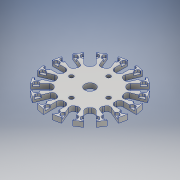
# Autodesk Inventor part: plate1_3mm_m6collet
Saved by Autodesk Inventor 2018 (Build 220112000, 112)
## iProperties
Created: 2017-08-17
Part Number: plate1_3mm_m6collet
Material: Aluminum 6061
Document SubType Name: Modeling
Designer: steve
Density: 2.7 g/cm^3
Appearance: Aluminum - Flat
Mass: 8.83202 g
Surface Area: 37.957 cm^2
Volume: 3.27112 cm^3
Author: steve
Autodesk Inventor part; units mm, degrees
note: some values were not read from the file. Chosen so that the rebuilt part matches the saved one: direction of "Hole3".
ref_plane "YZ Plane" through (0, 0, 0) normal (1, 0, 0) x (0, 1, 0)
ref_plane "XZ Plane" through (0, 0, 0) normal (0, 1, 0) x (-1, 0, 0)
ref_plane "XY Plane" through (0, 0, 0) normal (0, 0, 1) x (1, 0, 0)
sketch "Sketch1" plane through (0, 0, 0) normal (0, 0, 1) x (1, 0, 0)
  circle A0 centre (0, 0) radius 25
  dimension "wheel_border" = 50
  constraints: 1 centre point, 1 coincident
  measures "wheel_border" diameter of A0
extrude "Extrusion1" add sketch "Sketch1" along normal blind 3
sketch "Sketch4" plane through (0, 0, 3) normal (0, 0, 1) x (1, 0, 0)
  line L0 (-35, 0) -> (35, 0) construction
  line L1 (0, -35) -> (0, 35) construction
  line L2 (-11.282, 25) -> (10.768, 25) construction
  line L3 (-11.9075, 22.5) -> (11.2763, 22.5) construction
  circle A0 centre (0, 0) radius 25 construction
  line L4 (4.075, 20.9625) -> (-4.075, 20.9625) construction
  line L5 (-4.075, 20.9625) -> (-4.075, 24.0375) construction
  line L6 (-4.075, 24.0375) -> (4.075, 24.0375) construction
  line L7 (4.075, 24.0375) -> (4.075, 20.9625) construction
  line L8 (4.075, 20.9625) -> (-4.075, 24.0375) construction
  line L9 (-4.075, 20.9625) -> (4.075, 24.0375) construction
  line L10 (4.075, 20.9625) -> (-4.075, 20.9625)
  line L11 (-4.075, 20.9625) -> (-4.075, 24.0375)
  line L12 (-4.075, 24.0375) -> (4.075, 24.0375)
  line L13 (4.075, 24.0375) -> (4.075, 20.9625)
  line L14 (4.075, 20.9625) -> (-4.075, 24.0375) construction
  line L15 (-4.075, 20.9625) -> (4.075, 24.0375) construction
  point P0 (0, 22.5)
  dimension "d23" = 2.5
  dimension "d24" = 3.075
  dimension "d25" = 8.15
  constraints: 28 end point, 4 horizontal, 4 midpoint, 4 parallel, 2 perpendicular, 2 point on line, 1 tangent
  measures "d23" distance between parallel lines of L3 L2
  measures "d24" distance of L6.end L4.start
  measures "d25" distance of L4.start L4.end
extrude "Extrusion4" cut sketch "Sketch4" against normal blind 1.5
sketch "Sketch5" plane through (0, 0, 3) normal (0, 0, 1) x (1, 0, 0)
  line L0 (-4.075, 20.9625) -> (-4.075, 24.0375) construction
  line L1 (4.075, 20.9625) -> (-4.075, 20.9625) construction
  line L2 (4.075, 24.0375) -> (4.075, 20.9625) construction
  line L3 (-4.075, 24.0375) -> (4.075, 24.0375) construction
  line L4 (-35, 0) -> (35, 0) construction
  line L5 (0, -36.2) -> (0, 42.2) construction
  line L6 (-4.075, 22.5) -> (4.075, 22.5) construction
  line L7 (4.075, 24.0375) -> (4.075, 20.9625) construction
  line L8 (2.575, 15) -> (-2.575, 15)
  line L9 (-2.575, 15) -> (-2.575, 30)
  line L10 (-2.575, 30) -> (2.575, 30)
  line L11 (2.575, 30) -> (2.575, 15)
  line L12 (2.575, 15) -> (-2.575, 30) construction
  line L13 (-2.575, 15) -> (2.575, 30) construction
  point P0 (0, 0)
  point P1 (0, 22.5)
  dimension "d28" = 15
  dimension "d29" = 5.15
  constraints: 14 end point, 5 midpoint, 2 parallel, 1 horizontal, 1 perpendicular
  measures "d28" distance of L10.end L8.start
  measures "d29" distance of L8.start L8.end
extrude "Extrusion5" cut sketch "Sketch5" against normal blind 8.5
fillet "Fillet2" radius 2 2 edges at (-2.575, 15, 1.5) (2.575, 15, 1.5)
fillet "Fillet3" radius 1 4 edges at (-4.075, 24.0375, 2.25) (-4.075, 20.9625, 2.25) (4.075, 24.0375, 2.25) (4.075, 20.9625, 2.25)
pattern_circular "Circular Pattern1" count 16 over 360 about axis through (0, 0, 0) along (0, 0, 1) of "Extrusion4", "Extrusion5", "Fillet2", "Fillet3"
sketch "Sketch6" plane through (0, 0, 0) normal (0, 0, -1) x (-1, 0, 0)
  circle A0 centre (0, 0) radius 3
  dimension "d37" = 6
  constraints: 1 centre point, 1 coincident
  measures "d37" diameter of A0
sketch "Sketch9" plane through (0, 0, 0) normal (0, 0, -1) x (-1, 0, 0)
  circle A0 centre (0, 0) radius 22 construction
  line L0 (-6.8198, 23.1932) -> (-7.1372, 23.9596) construction
  arc A1 (-2.575, 24.867) -> (-7.1372, 23.9596) centre (0, 0) ccw construction
  line L1 (-2.575, 24.867) -> (-2.575, 24.0375) construction
  line L2 (-2.575, 24.0375) -> (-3.075, 24.0375) construction
  arc A2 (-3.075, 24.0375) -> (-4.075, 23.0375) centre (-3.075, 23.0375) ccw construction
  line L3 (-4.075, 23.0375) -> (-4.075, 21.9625) construction
  arc A3 (-4.075, 21.9625) -> (-3.075, 20.9625) centre (-3.075, 21.9625) ccw construction
  line L4 (-3.075, 20.9625) -> (-2.575, 20.9625) construction
  line L5 (-2.575, 20.9625) -> (-2.575, 17) construction
  arc A4 (-2.575, 17) -> (-0.575, 15) centre (-0.575, 17) ccw construction
  line L6 (-0.575, 15) -> (0.575, 15) construction
  arc A5 (0.575, 15) -> (2.575, 17) centre (0.575, 17) ccw construction
  line L7 (2.575, 17) -> (2.575, 20.9625) construction
  line L8 (2.575, 20.9625) -> (3.075, 20.9625) construction
  arc A6 (3.075, 20.9625) -> (4.075, 21.9625) centre (3.075, 21.9625) ccw construction
  line L9 (4.075, 21.9625) -> (4.075, 23.0375) construction
  arc A7 (4.075, 23.0375) -> (3.075, 24.0375) centre (3.075, 23.0375) ccw construction
  line L10 (3.075, 24.0375) -> (2.575, 24.0375) construction
  line L11 (2.575, 24.0375) -> (2.575, 24.867) construction
  arc A8 (7.1372, 23.9596) -> (2.575, 24.867) centre (0, 0) ccw construction
  line L12 (7.1372, 23.9596) -> (6.8198, 23.1932) construction
  line L13 (6.8198, 23.1932) -> (6.3578, 23.3845) construction
  arc A9 (6.3578, 23.3845) -> (5.0513, 22.8433) centre (5.9751, 22.4606) ccw construction
  line L14 (5.0513, 22.8433) -> (4.6399, 21.8501) construction
  arc A10 (4.6399, 21.8501) -> (5.1811, 20.5436) centre (5.5638, 21.4675) ccw construction
  line L15 (5.1811, 20.5436) -> (5.643, 20.3522) construction
  line L16 (5.643, 20.3522) -> (4.1266, 16.6914) construction
  arc A11 (4.1266, 16.6914) -> (5.209, 14.0782) centre (5.9744, 15.926) ccw construction
  line L17 (5.209, 14.0782) -> (6.2715, 13.6382) construction
  arc A12 (6.2715, 13.6382) -> (8.8846, 14.7205) centre (7.0368, 15.4859) ccw construction
  line L18 (8.8846, 14.7205) -> (10.401, 18.3814) construction
  line L19 (10.401, 18.3814) -> (10.8629, 18.1901) construction
  arc A13 (10.8629, 18.1901) -> (12.1695, 18.7313) centre (11.2456, 19.114) ccw construction
  line L20 (12.1695, 18.7313) -> (12.5809, 19.7244) construction
  arc A14 (12.5809, 19.7244) -> (12.0397, 21.031) centre (11.657, 20.1071) ccw construction
  line L21 (12.0397, 21.031) -> (11.5777, 21.2223) construction
  line L22 (11.5777, 21.2223) -> (11.8952, 21.9887) construction
  arc A15 (15.7628, 19.4044) -> (11.8952, 21.9887) centre (0, 0) ccw construction
  line L23 (15.7628, 19.4044) -> (15.1763, 18.8179) construction
  line L24 (15.1763, 18.8179) -> (14.8227, 19.1714) construction
  arc A16 (14.8227, 19.1714) -> (13.4085, 19.1714) centre (14.1156, 18.4643) ccw construction
  line L25 (13.4085, 19.1714) -> (12.6484, 18.4113) construction
  arc A17 (12.6484, 18.4113) -> (12.6484, 16.9971) centre (13.3555, 17.7042) ccw construction
  line L26 (12.6484, 16.9971) -> (13.0019, 16.6435) construction
  line L27 (13.0019, 16.6435) -> (10.2, 13.8416) construction
  arc A18 (10.2, 13.8416) -> (10.2, 11.0132) centre (11.6142, 12.4274) ccw construction
  line L28 (10.2, 11.0132) -> (11.0132, 10.2) construction
  arc A19 (11.0132, 10.2) -> (13.8416, 10.2) centre (12.4274, 11.6142) ccw construction
  line L29 (13.8416, 10.2) -> (16.6435, 13.0019) construction
  line L30 (16.6435, 13.0019) -> (16.9971, 12.6484) construction
  arc A20 (16.9971, 12.6484) -> (18.4113, 12.6484) centre (17.7042, 13.3555) ccw construction
  line L31 (18.4113, 12.6484) -> (19.1714, 13.4085) construction
  arc A21 (19.1714, 13.4085) -> (19.1714, 14.8227) centre (18.4643, 14.1156) ccw construction
  line L32 (19.1714, 14.8227) -> (18.8179, 15.1763) construction
  line L33 (18.8179, 15.1763) -> (19.4044, 15.7628) construction
  arc A22 (21.9887, 11.8952) -> (19.4044, 15.7628) centre (0, 0) ccw construction
  line L34 (21.9887, 11.8952) -> (21.2223, 11.5777) construction
  line L35 (21.2223, 11.5777) -> (21.031, 12.0397) construction
  arc A23 (21.031, 12.0397) -> (19.7244, 12.5809) centre (20.1071, 11.657) ccw construction
  line L36 (19.7244, 12.5809) -> (18.7313, 12.1695) construction
  arc A24 (18.7313, 12.1695) -> (18.1901, 10.8629) centre (19.114, 11.2456) ccw construction
  line L37 (18.1901, 10.8629) -> (18.3814, 10.401) construction
  line L38 (18.3814, 10.401) -> (14.7205, 8.8846) construction
  arc A25 (14.7205, 8.8846) -> (13.6382, 6.2715) centre (15.4859, 7.0368) ccw construction
  line L39 (13.6382, 6.2715) -> (14.0782, 5.209) construction
  arc A26 (14.0782, 5.209) -> (16.6914, 4.1266) centre (15.926, 5.9744) ccw construction
  line L40 (16.6914, 4.1266) -> (20.3522, 5.643) construction
  line L41 (20.3522, 5.643) -> (20.5436, 5.1811) construction
  arc A27 (20.5436, 5.1811) -> (21.8501, 4.6399) centre (21.4675, 5.5638) ccw construction
  line L42 (21.8501, 4.6399) -> (22.8433, 5.0513) construction
  arc A28 (22.8433, 5.0513) -> (23.3845, 6.3578) centre (22.4606, 5.9751) ccw construction
  line L43 (23.3845, 6.3578) -> (23.1932, 6.8198) construction
  line L44 (23.1932, 6.8198) -> (23.9596, 7.1372) construction
  arc A29 (24.867, 2.575) -> (23.9596, 7.1372) centre (0, 0) ccw construction
  line L45 (24.867, 2.575) -> (24.0375, 2.575) construction
  line L46 (24.0375, 2.575) -> (24.0375, 3.075) construction
  arc A30 (24.0375, 3.075) -> (23.0375, 4.075) centre (23.0375, 3.075) ccw construction
  line L47 (23.0375, 4.075) -> (21.9625, 4.075) construction
  arc A31 (21.9625, 4.075) -> (20.9625, 3.075) centre (21.9625, 3.075) ccw construction
  line L48 (20.9625, 3.075) -> (20.9625, 2.575) construction
  line L49 (20.9625, 2.575) -> (17, 2.575) construction
  arc A32 (17, 2.575) -> (15, 0.575) centre (17, 0.575) ccw construction
  line L50 (15, 0.575) -> (15, -0.575) construction
  arc A33 (15, -0.575) -> (17, -2.575) centre (17, -0.575) ccw construction
  line L51 (17, -2.575) -> (20.9625, -2.575) construction
  line L52 (20.9625, -2.575) -> (20.9625, -3.075) construction
  arc A34 (20.9625, -3.075) -> (21.9625, -4.075) centre (21.9625, -3.075) ccw construction
  line L53 (21.9625, -4.075) -> (23.0375, -4.075) construction
  arc A35 (23.0375, -4.075) -> (24.0375, -3.075) centre (23.0375, -3.075) ccw construction
  line L54 (24.0375, -3.075) -> (24.0375, -2.575) construction
  line L55 (24.0375, -2.575) -> (24.867, -2.575) construction
  arc A36 (23.9596, -7.1372) -> (24.867, -2.575) centre (0, 0) ccw construction
  line L56 (23.9596, -7.1372) -> (23.1932, -6.8198) construction
  line L57 (23.1932, -6.8198) -> (23.3845, -6.3578) construction
  arc A37 (23.3845, -6.3578) -> (22.8433, -5.0513) centre (22.4606, -5.9751) ccw construction
  line L58 (22.8433, -5.0513) -> (21.8501, -4.6399) construction
  arc A38 (21.8501, -4.6399) -> (20.5436, -5.1811) centre (21.4675, -5.5638) ccw construction
  line L59 (20.5436, -5.1811) -> (20.3522, -5.643) construction
  line L60 (20.3522, -5.643) -> (16.6914, -4.1266) construction
  arc A39 (16.6914, -4.1266) -> (14.0782, -5.209) centre (15.926, -5.9744) ccw construction
  line L61 (14.0782, -5.209) -> (13.6382, -6.2715) construction
  arc A40 (13.6382, -6.2715) -> (14.7205, -8.8846) centre (15.4859, -7.0368) ccw construction
  line L62 (14.7205, -8.8846) -> (18.3814, -10.401) construction
  line L63 (18.3814, -10.401) -> (18.1901, -10.8629) construction
  arc A41 (18.1901, -10.8629) -> (18.7313, -12.1695) centre (19.114, -11.2456) ccw construction
  line L64 (18.7313, -12.1695) -> (19.7244, -12.5809) construction
  arc A42 (19.7244, -12.5809) -> (21.031, -12.0397) centre (20.1071, -11.657) ccw construction
  line L65 (21.031, -12.0397) -> (21.2223, -11.5777) construction
  line L66 (21.2223, -11.5777) -> (21.9887, -11.8952) construction
  arc A43 (19.4044, -15.7628) -> (21.9887, -11.8952) centre (0, 0) ccw construction
  line L67 (19.4044, -15.7628) -> (18.8179, -15.1763) construction
  line L68 (18.8179, -15.1763) -> (19.1714, -14.8227) construction
  arc A44 (19.1714, -14.8227) -> (19.1714, -13.4085) centre (18.4643, -14.1156) ccw construction
  line L69 (19.1714, -13.4085) -> (18.4113, -12.6484) construction
  arc A45 (18.4113, -12.6484) -> (16.9971, -12.6484) centre (17.7042, -13.3555) ccw construction
  line L70 (16.9971, -12.6484) -> (16.6435, -13.0019) construction
  line L71 (16.6435, -13.0019) -> (13.8416, -10.2) construction
  arc A46 (13.8416, -10.2) -> (11.0132, -10.2) centre (12.4274, -11.6142) ccw construction
  line L72 (11.0132, -10.2) -> (10.2, -11.0132) construction
  arc A47 (10.2, -11.0132) -> (10.2, -13.8416) centre (11.6142, -12.4274) ccw construction
  line L73 (10.2, -13.8416) -> (13.0019, -16.6435) construction
  line L74 (13.0019, -16.6435) -> (12.6484, -16.9971) construction
  arc A48 (12.6484, -16.9971) -> (12.6484, -18.4113) centre (13.3555, -17.7042) ccw construction
  line L75 (12.6484, -18.4113) -> (13.4085, -19.1714) construction
  arc A49 (13.4085, -19.1714) -> (14.8227, -19.1714) centre (14.1156, -18.4643) ccw construction
  line L76 (14.8227, -19.1714) -> (15.1763, -18.8179) construction
  line L77 (15.1763, -18.8179) -> (15.7628, -19.4044) construction
  arc A50 (11.8952, -21.9887) -> (15.7628, -19.4044) centre (0, 0) ccw construction
  line L78 (11.8952, -21.9887) -> (11.5777, -21.2223) construction
  line L79 (11.5777, -21.2223) -> (12.0397, -21.031) construction
  arc A51 (12.0397, -21.031) -> (12.5809, -19.7244) centre (11.657, -20.1071) ccw construction
  line L80 (12.5809, -19.7244) -> (12.1695, -18.7313) construction
  arc A52 (12.1695, -18.7313) -> (10.8629, -18.1901) centre (11.2456, -19.114) ccw construction
  line L81 (10.8629, -18.1901) -> (10.401, -18.3814) construction
  line L82 (10.401, -18.3814) -> (8.8846, -14.7205) construction
  arc A53 (8.8846, -14.7205) -> (6.2715, -13.6382) centre (7.0368, -15.4859) ccw construction
  line L83 (6.2715, -13.6382) -> (5.209, -14.0782) construction
  arc A54 (5.209, -14.0782) -> (4.1266, -16.6914) centre (5.9744, -15.926) ccw construction
  line L84 (4.1266, -16.6914) -> (5.643, -20.3522) construction
  line L85 (5.643, -20.3522) -> (5.1811, -20.5436) construction
  arc A55 (5.1811, -20.5436) -> (4.6399, -21.8501) centre (5.5638, -21.4675) ccw construction
  line L86 (4.6399, -21.8501) -> (5.0513, -22.8433) construction
  arc A56 (5.0513, -22.8433) -> (6.3578, -23.3845) centre (5.9751, -22.4606) ccw construction
  line L87 (6.3578, -23.3845) -> (6.8198, -23.1932) construction
  line L88 (6.8198, -23.1932) -> (7.1372, -23.9596) construction
  arc A57 (2.575, -24.867) -> (7.1372, -23.9596) centre (0, 0) ccw construction
  line L89 (2.575, -24.867) -> (2.575, -24.0375) construction
  line L90 (2.575, -24.0375) -> (3.075, -24.0375) construction
  arc A58 (3.075, -24.0375) -> (4.075, -23.0375) centre (3.075, -23.0375) ccw construction
  line L91 (4.075, -23.0375) -> (4.075, -21.9625) construction
  arc A59 (4.075, -21.9625) -> (3.075, -20.9625) centre (3.075, -21.9625) ccw construction
  line L92 (3.075, -20.9625) -> (2.575, -20.9625) construction
  line L93 (2.575, -20.9625) -> (2.575, -17) construction
  arc A60 (2.575, -17) -> (0.575, -15) centre (0.575, -17) ccw construction
  line L94 (0.575, -15) -> (-0.575, -15) construction
  arc A61 (-0.575, -15) -> (-2.575, -17) centre (-0.575, -17) ccw construction
  line L95 (-2.575, -17) -> (-2.575, -20.9625) construction
  line L96 (-2.575, -20.9625) -> (-3.075, -20.9625) construction
  arc A62 (-3.075, -20.9625) -> (-4.075, -21.9625) centre (-3.075, -21.9625) ccw construction
  line L97 (-4.075, -21.9625) -> (-4.075, -23.0375) construction
  arc A63 (-4.075, -23.0375) -> (-3.075, -24.0375) centre (-3.075, -23.0375) ccw construction
  line L98 (-3.075, -24.0375) -> (-2.575, -24.0375) construction
  line L99 (-2.575, -24.0375) -> (-2.575, -24.867) construction
  arc A64 (-7.1372, -23.9596) -> (-2.575, -24.867) centre (0, 0) ccw construction
  line L100 (-7.1372, -23.9596) -> (-6.8198, -23.1932) construction
  line L101 (-6.8198, -23.1932) -> (-6.3578, -23.3845) construction
  arc A65 (-6.3578, -23.3845) -> (-5.0513, -22.8433) centre (-5.9751, -22.4606) ccw construction
  line L102 (-5.0513, -22.8433) -> (-4.6399, -21.8501) construction
  arc A66 (-4.6399, -21.8501) -> (-5.1811, -20.5436) centre (-5.5638, -21.4675) ccw construction
  line L103 (-5.1811, -20.5436) -> (-5.643, -20.3522) construction
  line L104 (-5.643, -20.3522) -> (-4.1266, -16.6914) construction
  arc A67 (-4.1266, -16.6914) -> (-5.209, -14.0782) centre (-5.9744, -15.926) ccw construction
  line L105 (-5.209, -14.0782) -> (-6.2715, -13.6382) construction
  arc A68 (-6.2715, -13.6382) -> (-8.8846, -14.7205) centre (-7.0368, -15.4859) ccw construction
  line L106 (-8.8846, -14.7205) -> (-10.401, -18.3814) construction
  line L107 (-10.401, -18.3814) -> (-10.8629, -18.1901) construction
  arc A69 (-10.8629, -18.1901) -> (-12.1695, -18.7313) centre (-11.2456, -19.114) ccw construction
  line L108 (-12.1695, -18.7313) -> (-12.5809, -19.7244) construction
  arc A70 (-12.5809, -19.7244) -> (-12.0397, -21.031) centre (-11.657, -20.1071) ccw construction
  line L109 (-12.0397, -21.031) -> (-11.5777, -21.2223) construction
  line L110 (-11.5777, -21.2223) -> (-11.8952, -21.9887) construction
  arc A71 (-15.7628, -19.4044) -> (-11.8952, -21.9887) centre (0, 0) ccw construction
  line L111 (-15.7628, -19.4044) -> (-15.1763, -18.8179) construction
  line L112 (-15.1763, -18.8179) -> (-14.8227, -19.1714) construction
  arc A72 (-14.8227, -19.1714) -> (-13.4085, -19.1714) centre (-14.1156, -18.4643) ccw construction
  line L113 (-13.4085, -19.1714) -> (-12.6484, -18.4113) construction
  arc A73 (-12.6484, -18.4113) -> (-12.6484, -16.9971) centre (-13.3555, -17.7042) ccw construction
  line L114 (-12.6484, -16.9971) -> (-13.0019, -16.6435) construction
  line L115 (-13.0019, -16.6435) -> (-10.2, -13.8416) construction
  arc A74 (-10.2, -13.8416) -> (-10.2, -11.0132) centre (-11.6142, -12.4274) ccw construction
  line L116 (-10.2, -11.0132) -> (-11.0132, -10.2) construction
  arc A75 (-11.0132, -10.2) -> (-13.8416, -10.2) centre (-12.4274, -11.6142) ccw construction
  line L117 (-13.8416, -10.2) -> (-16.6435, -13.0019) construction
  line L118 (-16.6435, -13.0019) -> (-16.9971, -12.6484) construction
  arc A76 (-16.9971, -12.6484) -> (-18.4113, -12.6484) centre (-17.7042, -13.3555) ccw construction
  line L119 (-18.4113, -12.6484) -> (-19.1714, -13.4085) construction
  arc A77 (-19.1714, -13.4085) -> (-19.1714, -14.8227) centre (-18.4643, -14.1156) ccw construction
  line L120 (-19.1714, -14.8227) -> (-18.8179, -15.1763) construction
  line L121 (-18.8179, -15.1763) -> (-19.4044, -15.7628) construction
  arc A78 (-21.9887, -11.8952) -> (-19.4044, -15.7628) centre (0, 0) ccw construction
  line L122 (-21.9887, -11.8952) -> (-21.2223, -11.5777) construction
  line L123 (-21.2223, -11.5777) -> (-21.031, -12.0397) construction
  arc A79 (-21.031, -12.0397) -> (-19.7244, -12.5809) centre (-20.1071, -11.657) ccw construction
  line L124 (-19.7244, -12.5809) -> (-18.7313, -12.1695) construction
  arc A80 (-18.7313, -12.1695) -> (-18.1901, -10.8629) centre (-19.114, -11.2456) ccw construction
  line L125 (-18.1901, -10.8629) -> (-18.3814, -10.401) construction
  line L126 (-18.3814, -10.401) -> (-14.7205, -8.8846) construction
  arc A81 (-14.7205, -8.8846) -> (-13.6382, -6.2715) centre (-15.4859, -7.0368) ccw construction
  line L127 (-13.6382, -6.2715) -> (-14.0782, -5.209) construction
  arc A82 (-14.0782, -5.209) -> (-16.6914, -4.1266) centre (-15.926, -5.9744) ccw construction
  line L128 (-16.6914, -4.1266) -> (-20.3522, -5.643) construction
  line L129 (-20.3522, -5.643) -> (-20.5436, -5.1811) construction
  arc A83 (-20.5436, -5.1811) -> (-21.8501, -4.6399) centre (-21.4675, -5.5638) ccw construction
  line L130 (-21.8501, -4.6399) -> (-22.8433, -5.0513) construction
  arc A84 (-22.8433, -5.0513) -> (-23.3845, -6.3578) centre (-22.4606, -5.9751) ccw construction
  line L131 (-23.3845, -6.3578) -> (-23.1932, -6.8198) construction
  line L132 (-23.1932, -6.8198) -> (-23.9596, -7.1372) construction
  arc A85 (-24.867, -2.575) -> (-23.9596, -7.1372) centre (0, 0) ccw construction
  line L133 (-24.867, -2.575) -> (-24.0375, -2.575) construction
  line L134 (-24.0375, -2.575) -> (-24.0375, -3.075) construction
  arc A86 (-24.0375, -3.075) -> (-23.0375, -4.075) centre (-23.0375, -3.075) ccw construction
  line L135 (-23.0375, -4.075) -> (-21.9625, -4.075) construction
  arc A87 (-21.9625, -4.075) -> (-20.9625, -3.075) centre (-21.9625, -3.075) ccw construction
  line L136 (-20.9625, -3.075) -> (-20.9625, -2.575) construction
  line L137 (-20.9625, -2.575) -> (-17, -2.575) construction
  arc A88 (-17, -2.575) -> (-15, -0.575) centre (-17, -0.575) ccw construction
  line L138 (-15, -0.575) -> (-15, 0.575) construction
  arc A89 (-15, 0.575) -> (-17, 2.575) centre (-17, 0.575) ccw construction
  line L139 (-17, 2.575) -> (-20.9625, 2.575) construction
  line L140 (-20.9625, 2.575) -> (-20.9625, 3.075) construction
  arc A90 (-20.9625, 3.075) -> (-21.9625, 4.075) centre (-21.9625, 3.075) ccw construction
  line L141 (-21.9625, 4.075) -> (-23.0375, 4.075) construction
  arc A91 (-23.0375, 4.075) -> (-24.0375, 3.075) centre (-23.0375, 3.075) ccw construction
  line L142 (-24.0375, 3.075) -> (-24.0375, 2.575) construction
  line L143 (-24.0375, 2.575) -> (-24.867, 2.575) construction
  arc A92 (-23.9596, 7.1372) -> (-24.867, 2.575) centre (0, 0) ccw construction
  line L144 (-23.9596, 7.1372) -> (-23.1932, 6.8198) construction
  line L145 (-23.1932, 6.8198) -> (-23.3845, 6.3578) construction
  arc A93 (-23.3845, 6.3578) -> (-22.8433, 5.0513) centre (-22.4606, 5.9751) ccw construction
  line L146 (-22.8433, 5.0513) -> (-21.8501, 4.6399) construction
  arc A94 (-21.8501, 4.6399) -> (-20.5436, 5.1811) centre (-21.4675, 5.5638) ccw construction
  line L147 (-20.5436, 5.1811) -> (-20.3522, 5.643) construction
  line L148 (-20.3522, 5.643) -> (-16.6914, 4.1266) construction
  arc A95 (-16.6914, 4.1266) -> (-14.0782, 5.209) centre (-15.926, 5.9744) ccw construction
  line L149 (-14.0782, 5.209) -> (-13.6382, 6.2715) construction
  arc A96 (-13.6382, 6.2715) -> (-14.7205, 8.8846) centre (-15.4859, 7.0368) ccw construction
  line L150 (-14.7205, 8.8846) -> (-18.3814, 10.401) construction
  line L151 (-18.3814, 10.401) -> (-18.1901, 10.8629) construction
  arc A97 (-18.1901, 10.8629) -> (-18.7313, 12.1695) centre (-19.114, 11.2456) ccw construction
  line L152 (-18.7313, 12.1695) -> (-19.7244, 12.5809) construction
  arc A98 (-19.7244, 12.5809) -> (-21.031, 12.0397) centre (-20.1071, 11.657) ccw construction
  line L153 (-21.031, 12.0397) -> (-21.2223, 11.5777) construction
  line L154 (-21.2223, 11.5777) -> (-21.9887, 11.8952) construction
  arc A99 (-19.4044, 15.7628) -> (-21.9887, 11.8952) centre (0, 0) ccw construction
  line L155 (-19.4044, 15.7628) -> (-18.8179, 15.1763) construction
  line L156 (-18.8179, 15.1763) -> (-19.1714, 14.8227) construction
  arc A100 (-19.1714, 14.8227) -> (-19.1714, 13.4085) centre (-18.4643, 14.1156) ccw construction
  line L157 (-19.1714, 13.4085) -> (-18.4113, 12.6484) construction
  arc A101 (-18.4113, 12.6484) -> (-16.9971, 12.6484) centre (-17.7042, 13.3555) ccw construction
  line L158 (-16.9971, 12.6484) -> (-16.6435, 13.0019) construction
  line L159 (-16.6435, 13.0019) -> (-13.8416, 10.2) construction
  arc A102 (-13.8416, 10.2) -> (-11.0132, 10.2) centre (-12.4274, 11.6142) ccw construction
  line L160 (-11.0132, 10.2) -> (-10.2, 11.0132) construction
  arc A103 (-10.2, 11.0132) -> (-10.2, 13.8416) centre (-11.6142, 12.4274) ccw construction
  line L161 (-10.2, 13.8416) -> (-13.0019, 16.6435) construction
  line L162 (-13.0019, 16.6435) -> (-12.6484, 16.9971) construction
  arc A104 (-12.6484, 16.9971) -> (-12.6484, 18.4113) centre (-13.3555, 17.7042) ccw construction
  line L163 (-12.6484, 18.4113) -> (-13.4085, 19.1714) construction
  arc A105 (-13.4085, 19.1714) -> (-14.8227, 19.1714) centre (-14.1156, 18.4643) ccw construction
  line L164 (-14.8227, 19.1714) -> (-15.1763, 18.8179) construction
  line L165 (-15.1763, 18.8179) -> (-15.7628, 19.4044) construction
  arc A106 (-11.8952, 21.9887) -> (-15.7628, 19.4044) centre (0, 0) ccw construction
  line L166 (-11.8952, 21.9887) -> (-11.5777, 21.2223) construction
  line L167 (-11.5777, 21.2223) -> (-12.0397, 21.031) construction
  arc A107 (-12.0397, 21.031) -> (-12.5809, 19.7244) centre (-11.657, 20.1071) ccw construction
  line L168 (-12.5809, 19.7244) -> (-12.1695, 18.7313) construction
  arc A108 (-12.1695, 18.7313) -> (-10.8629, 18.1901) centre (-11.2456, 19.114) ccw construction
  line L169 (-10.8629, 18.1901) -> (-10.401, 18.3814) construction
  line L170 (-10.401, 18.3814) -> (-8.8846, 14.7205) construction
  arc A109 (-8.8846, 14.7205) -> (-6.2715, 13.6382) centre (-7.0368, 15.4859) ccw construction
  line L171 (-6.2715, 13.6382) -> (-5.209, 14.0782) construction
  arc A110 (-5.209, 14.0782) -> (-4.1266, 16.6914) centre (-5.9744, 15.926) ccw construction
  line L172 (-4.1266, 16.6914) -> (-5.643, 20.3522) construction
  line L173 (-5.643, 20.3522) -> (-5.1811, 20.5436) construction
  arc A111 (-5.1811, 20.5436) -> (-4.6399, 21.8501) centre (-5.5638, 21.4675) ccw construction
  line L174 (-4.6399, 21.8501) -> (-5.0513, 22.8433) construction
  arc A112 (-5.0513, 22.8433) -> (-6.3578, 23.3845) centre (-5.9751, 22.4606) ccw construction
  line L175 (-6.3578, 23.3845) -> (-6.8198, 23.1932) construction
  line L176 (0, 0) -> (-38.1195, -7.5824) construction
  line L177 (37.6239, 0) -> (-50.7434, 0) construction
  point P0 (-21.5773, -4.292)
  point P1 (4.292, -21.5773)
  point P2 (21.5773, 4.292)
  point P3 (-4.292, 21.5773)
  dimension "d41" = 44
  dimension "d42" = 11.25
  dimension "d45" = 360
  constraints: 2 end point, 1 coincident, 1 point on line, 8 other
  measures "d42" angle of L177 L176
hole "Hole1" [suppressed]
sketch "Sketch10" plane through (0, 0, 3) normal (0, 0, 1) x (1, 0, 0)
  circle A0 centre (0, 0) radius 11 construction
  point P0 (11, 0)
  point P1 (0, 11)
  point P2 (-11, 0)
  point P3 (0, -11)
  dimension "d54" = 22
  constraints: 4 point on circle, 1 centre point, 1 coincident
  measures "d54" diameter of A0
hole "Hole2" at (11, 0, 3) at (0, 11, 3) at (-11, 0, 3) at (0, -11, 3) direction (0, 0, -1) diameter 2.459 end through all thread size "M3x0.5" class "6H" standard "ISO Metric profile"
hole "Hole3" at (0, 0, 0) direction (0, 0, 1) diameter 6.21 end up to surface
equation "\"d23\" = axis_to_border"
equation "\"d24\" = axis_w + 0.5 * fit_tol"
equation "\"d29\" = 2 * washer_w + bearing_w + fit_tol"
equation "\"fit_tol\" = 0.15"
equation "\"axis_w\" = 3"
equation "\"bearing_w\" = 4"
equation "\"washer_w\" = 0.5"
equation "\"bearing_l\" = 12"
equation "\"axis_to_border\" = 2.5"
body "Solid1"
